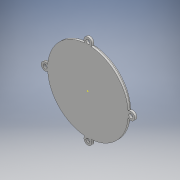
# Autodesk Inventor part: tapa
Saved by Autodesk Inventor 2018 (Build 220112000, 112)
## iProperties
Created: 2019-01-29
Part Number: tapa
Material: Generic
Document SubType Name: Modeling
Designer: Estudiante
Density: 1 g/cm^3
Appearance: Default
Author: Estudiante
Autodesk Inventor part; units mm, degrees
ref_plane "YZ Plane" through (0, 0, 0) normal (1, 0, 0) x (0, 1, 0)
ref_plane "XZ Plane" through (0, 0, 0) normal (0, 1, 0) x (-1, 0, 0)
ref_plane "XY Plane" through (0, 0, 0) normal (0, 0, 1) x (1, 0, 0)
sketch "Sketch1" plane through (0, 0, 0) normal (0, 1, 0) x (-1, 0, 0)
  arc A0 (18.9984, 0.2445) -> (18.9984, -0.2445) centre (0, 0) ccw
  circle A1 centre (0, 20.974) radius 0.987
  circle A2 centre (0, -20.974) radius 0.987
  arc A3 (18.9984, 0.2445) -> (18.9984, -0.2445) centre (0, 0) ccw
  arc A4 (18.9984, 0.2445) -> (18.9984, -0.2445) centre (20.9573, 0) ccw
  circle A5 centre (20.9573, 0) radius 0.987
  circle A6 centre (-21.0021, 0) radius 0.987
  arc A7 (-1.4939, 19.6837) -> (-19.6854, 1.4707) centre (0, 0) ccw
  arc A8 (-19.6854, 1.4707) -> (-19.6854, -1.4707) centre (-21.0021, 0) ccw
  arc A9 (-19.6854, -1.4707) -> (-1.4939, -19.6837) centre (0, 0) ccw
  arc A10 (-1.4939, -19.6837) -> (1.4939, -19.6837) centre (0, -20.974) ccw
  arc A11 (1.4939, -19.6837) -> (19.6826, -1.5074) centre (0, 0) ccw
  arc A12 (19.6826, -1.5074) -> (19.6826, 1.5074) centre (20.9573, 0) ccw
  arc A13 (19.6826, 1.5074) -> (1.4939, 19.6837) centre (0, 0) ccw
  arc A14 (1.4939, 19.6837) -> (-1.4939, 19.6837) centre (0, 20.974) ccw
  dimension "d0" = 19
  constraints: 22 point on circle, 15 centre point
  measures "d0" radius of A0
extrude "Extrusion1" add sketch "Sketch1" along normal blind 1
sketch "Sketch2" plane through (0, 1, 0) normal (0, 1, 0) x (1, 0, 0)
  arc A0 (-18.9984, -0.2445) -> (-18.9984, 0.2445) centre (0, 0) ccw projected
  arc A1 (-18.9984, -0.2445) -> (-18.9984, 0.2445) centre (-20.9573, 0) ccw projected
  arc A2 (-18.9984, -0.2445) -> (-18.9984, 0.2445) centre (0, 0) ccw projected
  circle A3 centre (-20.9573, 0) radius 0.987 projected
  circle A4 centre (0, 20.974) radius 0.987 projected
  circle A5 centre (21.0021, 0) radius 0.987 projected
  circle A6 centre (0, -20.974) radius 0.987 projected
  arc A7 (1.4939, -19.6837) -> (19.6854, -1.4707) centre (0, 0) ccw projected
  arc A8 (19.6854, -1.4707) -> (19.6854, 1.4707) centre (21.0021, 0) ccw projected
  arc A9 (19.6854, 1.4707) -> (1.4939, 19.6837) centre (0, 0) ccw projected
  arc A10 (1.4939, 19.6837) -> (-1.4939, 19.6837) centre (0, 20.974) ccw projected
  arc A11 (-1.4939, 19.6837) -> (-19.6826, 1.5074) centre (0, 0) ccw projected
  arc A12 (-19.6826, 1.5074) -> (-19.6826, -1.5074) centre (-20.9573, 0) ccw projected
  arc A13 (-19.6826, -1.5074) -> (-1.4939, -19.6837) centre (0, 0) ccw projected
  arc A14 (-1.4939, -19.6837) -> (1.4939, -19.6837) centre (0, -20.974) ccw projected
extrude "Extrusion2" add sketch "Sketch2" along normal mid plane 2 contours A1 A0
sketch "Sketch3" plane through (0, 0, 0) normal (0, -1, 0) x (1, 0, 0)
  point P0 (0, 0)
sketch "Sketch4" plane through (0, 2, 0) normal (0, 1, 0) x (1, 0, 0)
  arc A0 (-18.9984, -0.2445) -> (-18.9984, 0.2445) centre (0, 0) ccw projected
  circle A1 centre (0, 0) radius 18
  dimension "d5" = 36
  constraints: 1 centre point, 1 coincident
  measures "d5" diameter of A1
extrude "Extrusion3" cut sketch "Sketch4" against normal blind 1
body "Solid1"
